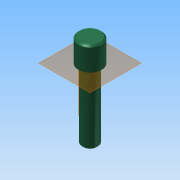
# Autodesk Inventor part: Ось
Saved by Autodesk Inventor 2013 (Build 170138000, 138)
## iProperties
Created: 2018-03-31
Part Number: Ось
Material: Типовые
Document SubType Name: Modeling
Designer: User
Density: 1 g/cm^3
Author: User
Autodesk Inventor part; units mm, degrees
ref_plane "YZ Plane" through (0, 0, 0) normal (1, 0, 0) x (0, 1, 0)
ref_plane "XZ Plane" through (0, 0, 0) normal (0, 1, 0) x (-1, 0, 0)
ref_plane "XY Plane" through (0, 0, 0) normal (0, 0, 1) x (1, 0, 0)
ref_plane "РабПлоскость1" through (0, 0, 0) normal (0, 0, 1) x (1, 0, 0)
sketch "Эскиз1" plane through (0, 0, 0) normal (0, 0, 1) x (1, 0, 0)
  circle A0 centre (0, 0) radius 10
  dimension "d0" = 20
  constraints: 1 centre point, 1 coincident
  measures "d0" diameter of A0
extrude "Выдавливание1" add sketch "Эскиз1" against normal blind 90
sketch "Эскиз2" plane through (0, 0, 0) normal (0, 0, 1) x (1, 0, 0)
  circle A0 centre (0, 0) radius 15
  dimension "d3" = 30
  constraints: 1 centre point, 1 coincident
  measures "d3" diameter of A0
extrude "Выдавливание2" add sketch "Эскиз2" along normal blind 30
chamfer "Фаска1" distance 2 angle 45 2 edges at (-15, 0, 30) (-10, 0, -90)
ref_plane "РабПлоскость2" through (-11.5, 3, -60) normal (1, 0, 0) x (0, 1, 0)
sketch "Эскиз3" plane through (-11.5, 3, -60) normal (1, 0, 0) x (0, 1, 0)
  line L0 (-18, 60) -> (12, 60) projected
  line L1 (12, 88) -> (-18, 88) projected
  line L2 (-13, 60) -> (7, 60) projected
  line L3 (-13, -28) -> (7, -28) projected
  line L4 (-3, 10) -> (-3, 10)
  line L5 (0, 13) -> (0, 47)
  line L6 (-3, 50) -> (-3, 50)
  line L7 (-6, 47) -> (-6, 13)
  line L8 (-6, 10) -> (0, 50) construction
  line L9 (0, 10) -> (-6, 50) construction
  arc A0 (0, 47) -> (-3, 50) centre (-3, 47) ccw
  arc A1 (-3, 50) -> (-6, 47) centre (-3, 47) ccw
  arc A2 (-3, 10) -> (0, 13) centre (-3, 13) ccw
  arc A3 (-6, 13) -> (-3, 10) centre (-3, 13) ccw
  point P0 (-3, 60)
  point P1 (-3, 30)
  dimension "d9" = 30
  dimension "d10" = 6
  dimension "d11" = 40
  dimension "d12" = 3
  constraints: 12 end point, 8 point on circle, 8 point on line, 8 tangent, 4 centre point, 3 equal radius, 2 midpoint, 2 parallel, 1 horizontal, 1 perpendicular
  measures "d9" distance from line of point (-3, 30) L0
  measures "d10" distance of L8.start L9.start
  measures "d11" distance between parallel lines of L4 L6
  measures "d12" radius of A0
extrude "Выдавливание3" cut sketch "Эскиз3" along normal blind 6
